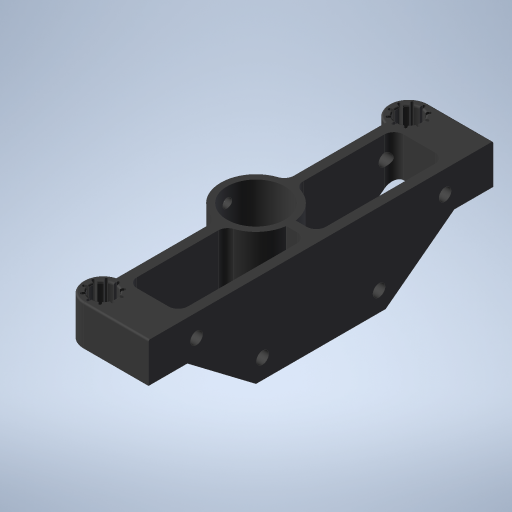
# Autodesk Inventor part: Arm Base stand
Saved by Autodesk Inventor 2024 (Build 280153000, 153)
## iProperties
Created: 2024-03-27
Part Number: Arm Base stand
Material: Generic
Document SubType Name: Modeling
Designer: drew
Density: 1 g/cm^3
Appearance: Default
Author: drew
Autodesk Inventor part; units mm, degrees
ref_plane "YZ Plane" through (0, 0, 0) normal (1, 0, 0) x (0, 1, 0)
ref_plane "XZ Plane" through (0, 0, 0) normal (0, 1, 0) x (-1, 0, 0)
ref_plane "XY Plane" through (0, 0, 0) normal (0, 0, 1) x (1, 0, 0)
sketch "Sketch1" plane through (0, 0, 0) normal (0, 1, 0) x (-1, 0, 0)
  circle A0 centre (0, 0) radius 11.43
  line L0 (-18.025, 21.2) -> (18.025, 21.2)
  line L1 (21.2, 18.025) -> (21.2, -18.025)
  line L2 (18.025, -21.2) -> (-18.025, -21.2)
  line L3 (-21.2, -18.025) -> (-21.2, 18.025)
  line L4 (-21.2, 21.2) -> (21.2, -21.2) construction
  line L5 (21.2, 21.2) -> (-21.2, -21.2) construction
  line L6 (21.2, 0) -> (-21.2, 0) construction
  line L7 (0, -21.2) -> (0, 21.2) construction
  circle A1 centre (15.5, -15.5) radius 1.6
  circle A2 centre (15.5, 15.5) radius 1.6
  circle A3 centre (-15.5, 15.5) radius 1.6
  circle A4 centre (-15.5, -15.5) radius 1.6
  arc A5 (21.2, 18.025) -> (18.025, 21.2) centre (18.025, 18.025) ccw
  arc A6 (18.025, -21.2) -> (21.2, -18.025) centre (18.025, -18.025) ccw
  arc A7 (-21.2, -18.025) -> (-18.025, -21.2) centre (-18.025, -18.025) ccw
  arc A8 (-18.025, 21.2) -> (-21.2, 18.025) centre (-18.025, 18.025) ccw
  dimension "d0" = 22.86
  dimension "d2" = 42.4
  dimension "d3" = 3.2
  dimension "d4" = 31
  dimension "d7" = 360
  dimension "d9" = 3.175
  constraints: 16 end point, 9 centre point, 9 point on line, 8 point on circle, 8 tangent, 6 midpoint, 3 equal radius, 2 parallel, 2 perpendicular, 1 coincident, 1 horizontal, 9 other
  measures "d0" diameter of A0
  measures "d2" distance of L4.end L5.end
  measures "d3" diameter of A1
  measures "d4" diameter of A1.centre L6
  measures "d9" radius of A5
extrude "Extrusion1" add sketch "Sketch1" along normal blind 2
sketch "Sketch2" plane through (0, 2, 0) normal (0, 1, 0) x (1, 0, 0)
  line L0 (18.025, 21.2) -> (-18.025, 21.2) projected
  arc A0 (-18.025, 21.2) -> (-21.2, 18.025) centre (-18.025, 18.025) ccw projected
  line L1 (-21.2, 18.025) -> (-21.2, -18.025) projected
  arc A1 (-21.2, -18.025) -> (-18.025, -21.2) centre (-18.025, -18.025) ccw projected
  line L2 (-18.025, -21.2) -> (18.025, -21.2) projected
  arc A2 (18.025, -21.2) -> (21.2, -18.025) centre (18.025, -18.025) ccw projected
  line L3 (21.2, -18.025) -> (21.2, 18.025) projected
  arc A3 (21.2, 18.025) -> (18.025, 21.2) centre (18.025, 18.025) ccw projected
  circle A4 centre (0, 0) radius 11.43 projected
  circle A5 centre (-15.5, 15.5) radius 1.6 projected
  circle A6 centre (-15.5, -15.5) radius 1.6 projected
  circle A7 centre (15.5, -15.5) radius 1.6 projected
  circle A8 centre (15.5, 15.5) radius 1.6 projected
  circle A9 centre (-15.5, -15.5) radius 4.6
  circle A10 centre (-15.5, 15.5) radius 4.6
  circle A11 centre (15.5, 15.5) radius 4.6
  circle A12 centre (15.5, -15.5) radius 4.6
  circle A13 centre (0, 0) radius 9.5
  dimension "d12" = 3
  dimension "d13" = 3
  dimension "d14" = 3
  dimension "d15" = 3
  dimension "d16" = 19
  constraints: 5 centre point, 1 coincident
  measures "d12" radial gap between concentric circles of A6 A9
  measures "d13" radial gap between concentric circles of A5 A10
  measures "d14" radial gap between concentric circles of A8 A11
  measures "d15" radial gap between concentric circles of A7 A12
  measures "d16" diameter of A13
extrude "Extrusion2" add sketch "Sketch2" along normal blind 25 contours A3 L3 A2 L2 A1 L1 A0 L0 | A4
sketch "Sketch4" plane through (0, 27, 0) normal (0, 1, 0) x (1, 0, 0)
  circle A0 centre (0, 0) radius 9.5 projected
  circle A1 centre (-15.5, 15.5) radius 4.6 projected
  circle A2 centre (-15.5, -15.5) radius 4.6 projected
  circle A3 centre (15.5, 15.5) radius 4.6 projected
  circle A4 centre (15.5, -15.5) radius 1.6 projected
  circle A5 centre (15.5, -15.5) radius 4.6 projected
  circle A6 centre (0, -50) radius 4
  line L0 (0, 0) -> (-2.5737, 0) construction
  circle A7 centre (0, 50) radius 4
  circle A8 centre (0, -50) radius 6.35
  circle A9 centre (0, 50) radius 6.35
  arc A10 (-18.025, 21.2) -> (-21.2, 18.025) centre (-18.025, 18.025) ccw projected
  line L1 (-21.2, 18.025) -> (-21.2, -18.025) projected
  arc A11 (-21.2, -18.025) -> (-18.025, -21.2) centre (-18.025, -18.025) ccw projected
  line L2 (-18.025, -21.2) -> (18.025, -21.2) projected
  arc A12 (18.025, -21.2) -> (21.2, -18.025) centre (18.025, -18.025) ccw projected
  line L3 (21.2, -18.025) -> (21.2, 18.025) projected
  arc A13 (21.2, 18.025) -> (18.025, 21.2) centre (18.025, 18.025) ccw projected
  line L4 (18.025, 21.2) -> (-18.025, 21.2) projected
  circle A14 centre (0, 0) radius 9.5 projected
  circle A15 centre (15.5, -15.5) radius 4.6 projected
  circle A16 centre (15.5, 15.5) radius 4.6 projected
  circle A17 centre (-15.5, 15.5) radius 4.6 projected
  circle A18 centre (-15.5, -15.5) radius 4.6 projected
  line L5 (-5.7806, -52.6281) -> (-20.9153, -19.3391)
  line L6 (-20.9153, 19.3391) -> (-5.7806, 52.6281)
  arc A19 (-21.2, -18.025) -> (-18.025, -21.2) centre (-18.025, -18.025) ccw projected
  line L7 (0, -56.35) -> (21.2, -56.35)
  line L8 (21.2, -56.35) -> (21.2, 56.35)
  line L9 (21.2, 56.35) -> (0, 56.35)
  line L10 (21.2, -18.025) -> (21.2, 18.025) projected
  point P0 (21.2, 18.025)
  dimension "d19" = 8
  dimension "d20" = 50
  dimension "d21" = 12.7
  dimension "d22" = 12.7
  constraints: 12 end point, 6 point on circle, 6 tangent, 4 centre point, 3 horizontal, 2 coincident, 1 collinear, 1 point on line, 1 symmetric about line, 1 vertical alignment, 1 other
  measures "d19" diameter of A6
  measures "d20" distance of point (0, 0) A6.centre
  measures "d21" diameter of A8
  measures "d22" diameter of A9
extrude "Extrusion3" add sketch "Sketch4" along normal blind 3 contours A6 | A7 | A8 | A8 L5 A11 L2 A12 L8 L7 | A11 L1 A10 L4 A13 L3 A12 L2 | A13 L4 A10 L6 A9 L9 L8 | A9
sketch "Sketch5" plane through (0, 30, 0) normal (0, 1, 0) x (1, 0, 0)
  arc A0 (-5.7806, -52.6281) -> (0, -56.35) centre (0, -50) ccw projected
  arc A1 (0, 56.35) -> (-5.7806, 52.6281) centre (0, 50) ccw projected
  circle A2 centre (0, -50) radius 4
  circle A3 centre (0, 50) radius 4
  point P0 (0, 0)
  dimension "d25" = 8
  dimension "d26" = 8
  constraints: 2 centre point, 2 coincident
  measures "d25" diameter of A2
  measures "d26" diameter of A3
extrude "Extrusion4" cut sketch "Sketch5" against normal blind 3
sketch "Sketch6" plane through (0, 27, 0) normal (0, -1, 0) x (1, 0, 0)
  circle A0 centre (0, -50) radius 4 projected
  arc A1 (-5.7806, -52.6281) -> (0, -56.35) centre (0, -50) ccw projected
  circle A2 centre (0, -50) radius 6.35
  circle A3 centre (0, 50) radius 4 projected
  circle A4 centre (0, 50) radius 6.35
  arc A5 (0, 56.35) -> (-5.7806, 52.6281) centre (0, 50) ccw projected
  point P0 (0, 0)
  point P1 (0, -56.35)
  point P2 (-5.7806, -52.6281)
  constraints: 2 centre point, 2 coincident, 2 concentric
extrude "Extrusion5" add sketch "Sketch6" along normal blind 7
sketch "Sketch7" plane through (0, 20, 50) normal (0, -1, 0) x (1, 0, 0)
  circle A0 centre (0, 0) radius 6.35 projected
  circle A1 centre (0, -100) radius 6.35 projected
  point P0 (0, -50)
extrude "Extrusion6" add sketch "Sketch7" along normal blind 3
sketch "Sketch8" plane through (0, 17, 50) normal (0, -1, 0) x (1, 0, 0)
  circle A0 centre (0, 0) radius 6.35 projected
  line L0 (0, 5) -> (0, -5) construction
  line L1 (-0.5, 5) -> (-0.5, -5)
  line L2 (0.5, -5) -> (0.5, 5)
  arc A1 (0.5, 5) -> (-0.5, 5) centre (0, 5) ccw
  arc A2 (-0.5, -5) -> (0.5, -5) centre (0, -5) ccw
  line L3 (-2.9389, 4.0451) -> (2.9389, -4.0451) construction
  line L4 (-3.3434, 3.7512) -> (2.5344, -4.339)
  line L5 (3.3434, -3.7512) -> (-2.5344, 4.339)
  arc A3 (-2.5344, 4.339) -> (-3.3434, 3.7512) centre (-2.9389, 4.0451) ccw
  arc A4 (2.5344, -4.339) -> (3.3434, -3.7512) centre (2.9389, -4.0451) ccw
  line L6 (-4.7553, 1.5451) -> (4.7553, -1.5451) construction
  line L7 (-4.9098, 1.0696) -> (4.6008, -2.0206)
  line L8 (4.9098, -1.0696) -> (-4.6008, 2.0206)
  arc A5 (-4.6008, 2.0206) -> (-4.9098, 1.0696) centre (-4.7553, 1.5451) ccw
  arc A6 (4.6008, -2.0206) -> (4.9098, -1.0696) centre (4.7553, -1.5451) ccw
  line L9 (-4.7553, -1.5451) -> (4.7553, 1.5451) construction
  line L10 (-4.6008, -2.0206) -> (4.9098, 1.0696)
  line L11 (4.6008, 2.0206) -> (-4.9098, -1.0696)
  arc A7 (-4.9098, -1.0696) -> (-4.6008, -2.0206) centre (-4.7553, -1.5451) ccw
  arc A8 (4.9098, 1.0696) -> (4.6008, 2.0206) centre (4.7553, 1.5451) ccw
  line L12 (-2.9389, -4.0451) -> (2.9389, 4.0451) construction
  line L13 (-2.5344, -4.339) -> (3.3434, 3.7512)
  line L14 (2.5344, 4.339) -> (-3.3434, -3.7512)
  arc A9 (-3.3434, -3.7512) -> (-2.5344, -4.339) centre (-2.9389, -4.0451) ccw
  arc A10 (3.3434, 3.7512) -> (2.5344, 4.339) centre (2.9389, 4.0451) ccw
  line L15 (0, -5) -> (0, 5) construction
  line L16 (0.5, -5) -> (0.5, 5)
  line L17 (-0.5, 5) -> (-0.5, -5)
  arc A11 (-0.5, -5) -> (0.5, -5) centre (0, -5) ccw
  arc A12 (0.5, 5) -> (-0.5, 5) centre (0, 5) ccw
  line L18 (0, -50) -> (2.9389, -50)
  circle A13 centre (0, -100) radius 6.35
  line L19 (0, -105) -> (0, -95) construction
  line L20 (-0.5, -105) -> (-0.5, -95)
  line L21 (0.5, -95) -> (0.5, -105)
  arc A14 (-0.5, -105) -> (0.5, -105) centre (0, -105) ccw
  arc A15 (0.5, -95) -> (-0.5, -95) centre (0, -95) ccw
  line L22 (-2.9389, -104.0451) -> (2.9389, -95.9549) construction
  line L23 (-3.3434, -103.7512) -> (2.5344, -95.661)
  line L24 (3.3434, -96.2488) -> (-2.5344, -104.339)
  arc A16 (-3.3434, -103.7512) -> (-2.5344, -104.339) centre (-2.9389, -104.0451) ccw
  arc A17 (3.3434, -96.2488) -> (2.5344, -95.661) centre (2.9389, -95.9549) ccw
  line L25 (-4.7553, -101.5451) -> (4.7553, -98.4549) construction
  line L26 (-4.9098, -101.0696) -> (4.6008, -97.9794)
  line L27 (4.9098, -98.9304) -> (-4.6008, -102.0206)
  arc A18 (-4.9098, -101.0696) -> (-4.6008, -102.0206) centre (-4.7553, -101.5451) ccw
  arc A19 (4.9098, -98.9304) -> (4.6008, -97.9794) centre (4.7553, -98.4549) ccw
  line L28 (-4.7553, -98.4549) -> (4.7553, -101.5451) construction
  line L29 (-4.6008, -97.9794) -> (4.9098, -101.0696)
  line L30 (4.6008, -102.0206) -> (-4.9098, -98.9304)
  arc A20 (-4.6008, -97.9794) -> (-4.9098, -98.9304) centre (-4.7553, -98.4549) ccw
  arc A21 (4.6008, -102.0206) -> (4.9098, -101.0696) centre (4.7553, -101.5451) ccw
  line L31 (-2.9389, -95.9549) -> (2.9389, -104.0451) construction
  line L32 (-2.5344, -95.661) -> (3.3434, -103.7512)
  line L33 (2.5344, -104.339) -> (-3.3434, -96.2488)
  arc A22 (-2.5344, -95.661) -> (-3.3434, -96.2488) centre (-2.9389, -95.9549) ccw
  arc A23 (2.5344, -104.339) -> (3.3434, -103.7512) centre (2.9389, -104.0451) ccw
  line L34 (0, -95) -> (0, -105) construction
  line L35 (0.5, -95) -> (0.5, -105)
  line L36 (-0.5, -105) -> (-0.5, -95)
  arc A24 (0.5, -95) -> (-0.5, -95) centre (0, -95) ccw
  arc A25 (-0.5, -105) -> (0.5, -105) centre (0, -105) ccw
  point P0 (-0.5, -1.5388)
  point P1 (0.5, -1.5388)
  point P2 (1.309, -0.9511)
  point P3 (1.618, 0)
  point P4 (1.309, 0.9511)
  point P5 (0.5, 1.5388)
  point P6 (-0.5, 1.5388)
  point P7 (-1.309, 0.9511)
  point P8 (-1.618, 0)
  point P9 (-1.309, -0.9511)
  point P10 (-0.5, -101.5388)
  point P11 (-0.5, -105)
  point P12 (0.5, -105)
  point P13 (0.5, -101.5388)
  point P14 (1.309, -100.9511)
  point P15 (1.618, -100)
  point P16 (1.309, -99.0489)
  point P17 (0.5, -98.4612)
  point P18 (0.5, -95)
  point P19 (-0.5, -95)
  point P20 (-0.5, -98.4612)
  point P21 (-1.309, -99.0489)
  point P22 (-1.618, -100)
  point P23 (-1.309, -100.9511)
  dimension "d33" = 10
  dimension "d34" = 0.5
  dimension "d37" = 180
  constraints: 98 end point, 48 point on circle, 37 symmetric about line, 25 centre point, 4 tangent, 1 horizontal, 1 midpoint, 1 parallel, 1 vertical, 69 other
  measures "d33" distance of L0.start L0.end
  measures "d34" radius of A2
extrude "Extrusion7" cut sketch "Sketch8" against normal through all contours A1 L2 L14 L5 L1 | L5 L14 L8 L1 | L1 L8 L4 A3 L5 | L8 L14 L11 L1 | L1 L11 L4 L8 | L14 L2 L11 L5 | L5 L11 L8 L14 | L14 A10 L13 L11 L2 | L11 L14 L1 | L1 L14 L4 L11 | L8 L11 L14 | L4 L11 L7 A5 L8 | L11 L2 L8 L5 | L5 L8 L11 | L11 L13 L8 L2 | L14 L11 L8 L5 L2 L13 L10 L7 L4 L1 | L1 L4 L14 | L4 L14 L7 L11 | L8 L2 L5 | L8 L13 L5 L2 | L11 A8 L10 L8 L13 | L4 L7 L1 | L1 L7 L14 L4 | L7 L14 L10 A7 L11 | L5 L13 L2 | L8 L10 L5 L13 | L7 L4 L10 L1 | L1 L10 L14 L7 | L7 L10 L4 | L13 L5 L10 L2 | L2 L10 L13 | L8 A6 L7 L5 L10 | L10 L4 L13 L1 | L1 L13 A9 L14 L10 | L10 L7 L13 L4 | L10 L13 L7 | L10 L5 L7 L2 | L2 L7 L13 L10 | L13 L4 L2 A2 L1 | L13 L7 L2 L4 | L7 L5 A4 L4 L2 | L20 L24 L33 L21 A14 | L24 A16 L23 L27 L20 | L20 L27 L33 L24 | L27 L23 L30 L20 | L20 L30 L33 L27 | L33 L27 L30 L24 | L24 L30 L21 L33 | L21 L30 L32 A23 L33 | L30 L23 L33 L20 | L20 L33 L30 | L33 L30 L27 | L27 A18 L26 L30 L23 | L30 L27 L24 | L24 L27 L21 L30 | L21 L27 L32 L30 | L33 L23 L20 | L20 L23 L26 L29 L32 L21 L24 L27 L30 L33 | L30 L26 L33 L23 | L24 L21 L27 | L21 L24 L32 L27 | L32 L27 L29 A21 L30 | L23 L33 L26 L20 | L20 L26 L23 | L30 A20 L29 L33 L26 | L21 L32 L24 | L32 L24 L29 L27 | L26 L33 L29 L20 | L20 L29 L23 L26 | L23 L29 L26 | L32 L29 L21 | L21 L29 L24 L32 | L29 L24 L26 A19 L27 | L29 L33 A22 L32 L20 | L20 L32 L23 L29 | L23 L32 L26 L29 | L26 L32 L29 | L29 L32 L26 L21 | L21 L26 L24 L29 | L20 A15 L21 L23 L32 | L23 L21 L26 L32 | L21 L23 A17 L24 L26
ref_plane "Work Plane2" through (0, 0, 0) normal (1, 0, 0) x (0, 1, 0)
sketch "Sketch11" plane through (0, 0, 0) normal (1, 0, 0) x (0, 1, 0)
  line L0 (17, -43.65) -> (27, -43.65) projected
  line L1 (27, -52.6281) -> (27, -19.3391) projected
  line L2 (0, -21.2) -> (27, -21.2) projected
  line L3 (0, 21.2) -> (27, 21.2) projected
  line L4 (27, 19.3391) -> (27, 52.6281) projected
  line L5 (17, 43.65) -> (27, 43.65) projected
  line L6 (17, 43.65) -> (0, 21.2)
  line L7 (0, -21.2) -> (17, -43.65)
  line L8 (17, -43.65) -> (27, -43.65)
  line L9 (27, -43.65) -> (27, -44.15)
  line L10 (27, -44.15) -> (17, -44.15)
  line L11 (17, -44.15) -> (17, -43.65)
  line L12 (17, 43.65) -> (27, 43.65)
  line L13 (27, 43.65) -> (27, 44.15)
  line L14 (27, 44.15) -> (17, 44.15)
  line L15 (17, 44.15) -> (17, 43.65)
  point P0 (0, 0)
  dimension "d46" = 0.5
  dimension "d47" = 0.5
  constraints: 20 end point, 4 parallel, 2 horizontal, 2 perpendicular, 2 point on line
  measures "d46" distance between parallel lines of L0 L10
  measures "d47" distance between parallel lines of L5 L14
extrude "Extrusion9" add sketch "Sketch11" along normal mid plane 3
sketch "Sketch12" plane through (0, 30, 0) normal (0, 1, 0) x (1, 0, 0)
  line L0 (4.6008, -52.0206) -> (3.6199, -51.7019) projected
  arc A0 (2.7372, -52.9168) -> (3.6199, -51.7019) centre (0, -50) ccw projected
  line L1 (2.7372, -52.9168) -> (3.3434, -53.7512) projected
  arc A1 (2.5344, -54.339) -> (3.3434, -53.7512) centre (2.9389, -54.0451) ccw projected
  line L2 (2.5344, -54.339) -> (1.9282, -53.5046) projected
  arc A2 (0.5, -53.9686) -> (1.9282, -53.5046) centre (0, -50) ccw projected
  line L3 (0.5, -53.9686) -> (0.5, -55) projected
  arc A3 (-0.5, -55) -> (0.5, -55) centre (0, -55) ccw projected
  line L4 (-0.5, -55) -> (-0.5, -53.9686) projected
  arc A4 (-1.9282, -53.5046) -> (-0.5, -53.9686) centre (0, -50) ccw projected
  line L5 (-1.9282, -53.5046) -> (-2.5344, -54.339) projected
  arc A5 (-3.3434, -53.7512) -> (-2.5344, -54.339) centre (-2.9389, -54.0451) ccw projected
  line L6 (-3.3434, -53.7512) -> (-2.7372, -52.9168) projected
  arc A6 (-3.6199, -51.7019) -> (-2.7372, -52.9168) centre (0, -50) ccw projected
  line L7 (-3.6199, -51.7019) -> (-4.6008, -52.0206) projected
  arc A7 (-4.9098, -51.0696) -> (-4.6008, -52.0206) centre (-4.7553, -51.5451) ccw projected
  line L8 (-4.9098, -51.0696) -> (-3.9289, -50.7508) projected
  arc A8 (-3.9289, -49.2492) -> (-3.9289, -50.7508) centre (0, -50) ccw projected
  line L9 (-3.9289, -49.2492) -> (-4.9098, -48.9304) projected
  arc A9 (-4.6008, -47.9794) -> (-4.9098, -48.9304) centre (-4.7553, -48.4549) ccw projected
  line L10 (-4.6008, -47.9794) -> (-3.6199, -48.2981) projected
  arc A10 (-2.7372, -47.0832) -> (-3.6199, -48.2981) centre (0, -50) ccw projected
  line L11 (-2.7372, -47.0832) -> (-3.3434, -46.2488) projected
  arc A11 (-2.5344, -45.661) -> (-3.3434, -46.2488) centre (-2.9389, -45.9549) ccw projected
  line L12 (-2.5344, -45.661) -> (-1.9282, -46.4954) projected
  arc A12 (-0.5, -46.0314) -> (-1.9282, -46.4954) centre (0, -50) ccw projected
  line L13 (-0.5, -46.0314) -> (-0.5, -45) projected
  arc A13 (0.5, -45) -> (-0.5, -45) centre (0, -45) ccw projected
  line L14 (0.5, -45) -> (0.5, -46.0314) projected
  arc A14 (1.9282, -46.4954) -> (0.5, -46.0314) centre (0, -50) ccw projected
  line L15 (1.9282, -46.4954) -> (2.5344, -45.661) projected
  arc A15 (3.3434, -46.2488) -> (2.5344, -45.661) centre (2.9389, -45.9549) ccw projected
  line L16 (3.3434, -46.2488) -> (2.7372, -47.0832) projected
  arc A16 (3.6199, -48.2981) -> (2.7372, -47.0832) centre (0, -50) ccw projected
  line L17 (3.6199, -48.2981) -> (4.6008, -47.9794) projected
  arc A17 (4.9098, -48.9304) -> (4.6008, -47.9794) centre (4.7553, -48.4549) ccw projected
  line L18 (4.9098, -48.9304) -> (3.9289, -49.2492) projected
  arc A18 (3.9289, -50.7508) -> (3.9289, -49.2492) centre (0, -50) ccw projected
  line L19 (3.9289, -50.7508) -> (4.9098, -51.0696) projected
  arc A19 (4.6008, -52.0206) -> (4.9098, -51.0696) centre (4.7553, -51.5451) ccw projected
  line L20 (2.5344, 45.661) -> (1.9282, 46.4954) projected
  arc A20 (0.5, 46.0314) -> (1.9282, 46.4954) centre (0, 50) ccw projected
  line L21 (0.5, 46.0314) -> (0.5, 45) projected
  arc A21 (-0.5, 45) -> (0.5, 45) centre (0, 45) ccw projected
  line L22 (-0.5, 45) -> (-0.5, 46.0314) projected
  arc A22 (-1.9282, 46.4954) -> (-0.5, 46.0314) centre (0, 50) ccw projected
  line L23 (-1.9282, 46.4954) -> (-2.5344, 45.661) projected
  arc A23 (-3.3434, 46.2488) -> (-2.5344, 45.661) centre (-2.9389, 45.9549) ccw projected
  line L24 (-3.3434, 46.2488) -> (-2.7372, 47.0832) projected
  arc A24 (-3.6199, 48.2981) -> (-2.7372, 47.0832) centre (0, 50) ccw projected
  line L25 (-3.6199, 48.2981) -> (-4.6008, 47.9794) projected
  arc A25 (-4.9098, 48.9304) -> (-4.6008, 47.9794) centre (-4.7553, 48.4549) ccw projected
  line L26 (-4.9098, 48.9304) -> (-3.9289, 49.2492) projected
  arc A26 (-3.9289, 50.7508) -> (-3.9289, 49.2492) centre (0, 50) ccw projected
  line L27 (-3.9289, 50.7508) -> (-4.9098, 51.0696) projected
  arc A27 (-4.6008, 52.0206) -> (-4.9098, 51.0696) centre (-4.7553, 51.5451) ccw projected
  line L28 (-4.6008, 52.0206) -> (-3.6199, 51.7019) projected
  arc A28 (-2.7372, 52.9168) -> (-3.6199, 51.7019) centre (0, 50) ccw projected
  line L29 (-2.7372, 52.9168) -> (-3.3434, 53.7512) projected
  arc A29 (-2.5344, 54.339) -> (-3.3434, 53.7512) centre (-2.9389, 54.0451) ccw projected
  line L30 (-2.5344, 54.339) -> (-1.9282, 53.5046) projected
  arc A30 (-0.5, 53.9686) -> (-1.9282, 53.5046) centre (0, 50) ccw projected
  line L31 (-0.5, 53.9686) -> (-0.5, 55) projected
  arc A31 (0.5, 55) -> (-0.5, 55) centre (0, 55) ccw projected
  line L32 (0.5, 55) -> (0.5, 53.9686) projected
  arc A32 (1.9282, 53.5046) -> (0.5, 53.9686) centre (0, 50) ccw projected
  line L33 (1.9282, 53.5046) -> (2.5344, 54.339) projected
  arc A33 (3.3434, 53.7512) -> (2.5344, 54.339) centre (2.9389, 54.0451) ccw projected
  line L34 (3.3434, 53.7512) -> (2.7372, 52.9168) projected
  arc A34 (3.6199, 51.7019) -> (2.7372, 52.9168) centre (0, 50) ccw projected
  line L35 (3.6199, 51.7019) -> (4.6008, 52.0206) projected
  arc A35 (4.9098, 51.0696) -> (4.6008, 52.0206) centre (4.7553, 51.5451) ccw projected
  line L36 (4.9098, 51.0696) -> (3.9289, 50.7508) projected
  arc A36 (3.9289, 49.2492) -> (3.9289, 50.7508) centre (0, 50) ccw projected
  line L37 (3.9289, 49.2492) -> (4.9098, 48.9304) projected
  arc A37 (4.6008, 47.9794) -> (4.9098, 48.9304) centre (4.7553, 48.4549) ccw projected
  line L38 (4.6008, 47.9794) -> (3.6199, 48.2981) projected
  arc A38 (2.7372, 47.0832) -> (3.6199, 48.2981) centre (0, 50) ccw projected
  line L39 (2.7372, 47.0832) -> (3.3434, 46.2488) projected
  arc A39 (2.5344, 45.661) -> (3.3434, 46.2488) centre (2.9389, 45.9549) ccw projected
  arc A40 (-5.7806, -52.6281) -> (0, -56.35) centre (0, -50) ccw projected
  line L40 (0, -56.35) -> (21.2, -56.35) projected
  line L41 (21.2, -56.35) -> (21.2, 56.35) projected
  line L42 (21.2, 56.35) -> (0, 56.35) projected
  arc A41 (0, 56.35) -> (-5.7806, 52.6281) centre (0, 50) ccw projected
  line L43 (-5.7806, 52.6281) -> (-20.9153, 19.3391) projected
  arc A42 (-20.9153, 19.3391) -> (-21.2, 18.025) centre (-18.025, 18.025) ccw projected
  line L44 (-21.2, 18.025) -> (-21.2, -18.025) projected
  arc A43 (-21.2, -18.025) -> (-20.9153, -19.3391) centre (-18.025, -18.025) ccw projected
  line L45 (-20.9153, -19.3391) -> (-5.7806, -52.6281) projected
  circle A44 centre (15.5, -15.5) radius 4.6 projected
  circle A45 centre (15.5, 15.5) radius 4.6 projected
  circle A46 centre (-15.5, -15.5) radius 4.6 projected
  circle A47 centre (-15.5, 15.5) radius 4.6 projected
  circle A48 centre (0, 0) radius 9.5 projected
  line L46 (1.5, -43.8297) -> (1.5, -21.2) projected
  line L47 (-1.5, -21.2) -> (-1.5, -43.8297) projected
  line L48 (1.5, 21.2) -> (1.5, 43.8297) projected
  line L49 (-1.5, 43.8297) -> (-1.5, 21.2) projected
  circle A49 centre (0, 0) radius 11.5
  circle A50 centre (0, -50) radius 6.35
  circle A51 centre (0, 50) radius 6.35
  arc A52 (0, 56.35) -> (-5.7806, 52.6281) centre (0, 50) ccw projected
  line L50 (-1.5, -21.2) -> (-1.5, 21.2)
  line L51 (1.5, 21.2) -> (1.5, -21.2)
  point P0 (1.5, 11.4018)
  point P1 (1.5, -11.4018)
  point P2 (0, -56.35)
  point P3 (-5.7806, -52.6281)
  point P4 (-1.5, -11.4018)
  point P5 (-1.5, 11.4018)
  point P6 (-5.7806, 52.6281)
  dimension "d48" = 2
  constraints: 4 end point, 3 centre point, 2 coincident, 2 concentric, 1 parallel, 1 vertical
  measures "d48" radial gap between concentric circles of A48 A49
extrude "Extrusion10" cut sketch "Sketch12" against normal up to surface (28 mm away) contours L45 A43 L44 A42 L43 A51 L49 L50 A49 L47 A50 | A50 L46 L51 A49 L48 A51 L42 L41 L40
sketch "Sketch13" plane through (1.5, 0, 0) normal (1, 0, 0) x (0, 0, -1)
  circle A0 centre (0, 25.2375) radius 1.5
  circle A1 centre (0, 9.3625) radius 1.5
  line L0 (11.4018, 30) -> (-11.4018, 30) projected
  point P0 (0, 0)
  point P1 (0, 30)
  dimension "d51" = 3
  dimension "d52" = 3
  dimension "d53" = 4.7625
  dimension "d54" = 15.875
  constraints: 2 centre point, 2 vertical alignment, 1 midpoint
  measures "d51" diameter of A0
  measures "d52" diameter of A1
  measures "d53" distance of point (0, 30) A0.centre
  measures "d54" distance of A1.centre A0.centre
extrude "Extrusion11" cut sketch "Sketch13" against normal through all
sketch "Sketch15" plane through (21.2, 0, 18.025) normal (1, 0, 0) x (0, 0, -1)
  line L0 (-25.625, 17) -> (-3.175, 0) projected
  line L1 (-3.175, 2) -> (-3.175, 0) projected
  line L2 (-3.175, 2) -> (6.6232, 2) projected
  line L3 (6.6232, 30) -> (6.6232, 2) projected
  line L4 (-25.8047, 30) -> (6.6232, 30) projected
  line L5 (-25.8047, 17) -> (-25.8047, 30) projected
  line L6 (-25.8047, 17) -> (-25.625, 17) projected
  line L7 (39.225, 0) -> (39.225, 2) projected
  line L8 (39.225, 0) -> (61.675, 17) projected
  line L9 (61.675, 17) -> (61.8547, 17) projected
  line L10 (61.8547, 30) -> (61.8547, 17) projected
  line L11 (29.4268, 30) -> (61.8547, 30) projected
  line L12 (29.4268, 30) -> (29.4268, 2) projected
  line L13 (29.4268, 2) -> (39.225, 2) projected
  line L14 (6.6232, 30) -> (29.4268, 30)
  line L15 (39.225, 0) -> (-3.175, 0)
  line L16 (-38.325, 17) -> (-38.325, 30) projected
  line L17 (-25.8047, 30) -> (-38.325, 30)
  line L18 (-38.325, 30) -> (-38.325, 17)
  line L19 (-38.325, 17) -> (-25.8047, 17)
  line L20 (-25.8047, 17) -> (-25.8047, 30)
  line L21 (61.8547, 17) -> (74.375, 17) projected
  line L22 (61.8547, 30) -> (74.375, 30)
  line L23 (74.375, 30) -> (74.375, 17)
  line L24 (74.375, 17) -> (61.8547, 17)
  line L25 (61.8547, 17) -> (61.8547, 30)
  point P0 (18.025, 0)
  constraints: 20 end point, 5 parallel, 2 collinear, 2 horizontal, 2 perpendicular, 1 point on line
extrude "Extrusion12" add sketch "Sketch15" against normal blind 3
sketch "Sketch16" plane through (0, 30, 0) normal (0, 1, 0) x (1, 0, 0)
  line L0 (21.2, 56.35) -> (21.2, -56.35) projected
  line L1 (21.2, 56.35) -> (18.2, 56.35) projected
  line L2 (18.2, -56.35) -> (18.2, 56.35) projected
  line L3 (21.2, -56.35) -> (18.2, -56.35) projected
  arc A0 (1.5, 43.8297) -> (-1.5, 43.8297) centre (0, 50) ccw projected
  line L4 (-1.5, 43.8297) -> (-1.5, 11.4018) projected
  arc A1 (-1.5, 11.4018) -> (-1.5, -11.4018) centre (0, 0) ccw projected
  line L5 (-1.5, -11.4018) -> (-1.5, -43.8297) projected
  arc A2 (-1.5, -43.8297) -> (1.5, -43.8297) centre (0, -50) ccw projected
  line L6 (1.5, -43.8297) -> (1.5, -11.4018) projected
  arc A3 (1.5, -11.4018) -> (1.5, 11.4018) centre (0, 0) ccw projected
  line L7 (1.5, 11.4018) -> (1.5, 43.8297) projected
  line L8 (4.6008, -52.0206) -> (3.6199, -51.7019) projected
  arc A4 (2.7372, -52.9168) -> (3.6199, -51.7019) centre (0, -50) ccw projected
  line L9 (2.7372, -52.9168) -> (3.3434, -53.7512) projected
  arc A5 (2.5344, -54.339) -> (3.3434, -53.7512) centre (2.9389, -54.0451) ccw projected
  line L10 (2.5344, -54.339) -> (1.9282, -53.5046) projected
  arc A6 (0.5, -53.9686) -> (1.9282, -53.5046) centre (0, -50) ccw projected
  line L11 (0.5, -53.9686) -> (0.5, -55) projected
  arc A7 (-0.5, -55) -> (0.5, -55) centre (0, -55) ccw projected
  line L12 (-0.5, -55) -> (-0.5, -53.9686) projected
  arc A8 (-1.9282, -53.5046) -> (-0.5, -53.9686) centre (0, -50) ccw projected
  line L13 (-1.9282, -53.5046) -> (-2.5344, -54.339) projected
  arc A9 (-3.3434, -53.7512) -> (-2.5344, -54.339) centre (-2.9389, -54.0451) ccw projected
  line L14 (-3.3434, -53.7512) -> (-2.7372, -52.9168) projected
  arc A10 (-3.6199, -51.7019) -> (-2.7372, -52.9168) centre (0, -50) ccw projected
  line L15 (-3.6199, -51.7019) -> (-4.6008, -52.0206) projected
  arc A11 (-4.9098, -51.0696) -> (-4.6008, -52.0206) centre (-4.7553, -51.5451) ccw projected
  line L16 (-4.9098, -51.0696) -> (-3.9289, -50.7508) projected
  arc A12 (-3.9289, -49.2492) -> (-3.9289, -50.7508) centre (0, -50) ccw projected
  line L17 (-3.9289, -49.2492) -> (-4.9098, -48.9304) projected
  arc A13 (-4.6008, -47.9794) -> (-4.9098, -48.9304) centre (-4.7553, -48.4549) ccw projected
  line L18 (-4.6008, -47.9794) -> (-3.6199, -48.2981) projected
  arc A14 (-2.7372, -47.0832) -> (-3.6199, -48.2981) centre (0, -50) ccw projected
  line L19 (-2.7372, -47.0832) -> (-3.3434, -46.2488) projected
  arc A15 (-2.5344, -45.661) -> (-3.3434, -46.2488) centre (-2.9389, -45.9549) ccw projected
  line L20 (-2.5344, -45.661) -> (-1.9282, -46.4954) projected
  arc A16 (-0.5, -46.0314) -> (-1.9282, -46.4954) centre (0, -50) ccw projected
  line L21 (-0.5, -46.0314) -> (-0.5, -45) projected
  arc A17 (0.5, -45) -> (-0.5, -45) centre (0, -45) ccw projected
  line L22 (0.5, -45) -> (0.5, -46.0314) projected
  arc A18 (1.9282, -46.4954) -> (0.5, -46.0314) centre (0, -50) ccw projected
  line L23 (1.9282, -46.4954) -> (2.5344, -45.661) projected
  arc A19 (3.3434, -46.2488) -> (2.5344, -45.661) centre (2.9389, -45.9549) ccw projected
  line L24 (3.3434, -46.2488) -> (2.7372, -47.0832) projected
  arc A20 (3.6199, -48.2981) -> (2.7372, -47.0832) centre (0, -50) ccw projected
  line L25 (3.6199, -48.2981) -> (4.6008, -47.9794) projected
  arc A21 (4.9098, -48.9304) -> (4.6008, -47.9794) centre (4.7553, -48.4549) ccw projected
  line L26 (4.9098, -48.9304) -> (3.9289, -49.2492) projected
  arc A22 (3.9289, -50.7508) -> (3.9289, -49.2492) centre (0, -50) ccw projected
  line L27 (3.9289, -50.7508) -> (4.9098, -51.0696) projected
  arc A23 (4.6008, -52.0206) -> (4.9098, -51.0696) centre (4.7553, -51.5451) ccw projected
  line L28 (2.5344, 45.661) -> (1.9282, 46.4954) projected
  arc A24 (0.5, 46.0314) -> (1.9282, 46.4954) centre (0, 50) ccw projected
  line L29 (0.5, 46.0314) -> (0.5, 45) projected
  arc A25 (-0.5, 45) -> (0.5, 45) centre (0, 45) ccw projected
  line L30 (-0.5, 45) -> (-0.5, 46.0314) projected
  arc A26 (-1.9282, 46.4954) -> (-0.5, 46.0314) centre (0, 50) ccw projected
  line L31 (-1.9282, 46.4954) -> (-2.5344, 45.661) projected
  arc A27 (-3.3434, 46.2488) -> (-2.5344, 45.661) centre (-2.9389, 45.9549) ccw projected
  line L32 (-3.3434, 46.2488) -> (-2.7372, 47.0832) projected
  arc A28 (-3.6199, 48.2981) -> (-2.7372, 47.0832) centre (0, 50) ccw projected
  line L33 (-3.6199, 48.2981) -> (-4.6008, 47.9794) projected
  arc A29 (-4.9098, 48.9304) -> (-4.6008, 47.9794) centre (-4.7553, 48.4549) ccw projected
  line L34 (-4.9098, 48.9304) -> (-3.9289, 49.2492) projected
  arc A30 (-3.9289, 50.7508) -> (-3.9289, 49.2492) centre (0, 50) ccw projected
  line L35 (-3.9289, 50.7508) -> (-4.9098, 51.0696) projected
  arc A31 (-4.6008, 52.0206) -> (-4.9098, 51.0696) centre (-4.7553, 51.5451) ccw projected
  line L36 (-4.6008, 52.0206) -> (-3.6199, 51.7019) projected
  arc A32 (-2.7372, 52.9168) -> (-3.6199, 51.7019) centre (0, 50) ccw projected
  line L37 (-2.7372, 52.9168) -> (-3.3434, 53.7512) projected
  arc A33 (-2.5344, 54.339) -> (-3.3434, 53.7512) centre (-2.9389, 54.0451) ccw projected
  line L38 (-2.5344, 54.339) -> (-1.9282, 53.5046) projected
  arc A34 (-0.5, 53.9686) -> (-1.9282, 53.5046) centre (0, 50) ccw projected
  line L39 (-0.5, 53.9686) -> (-0.5, 55) projected
  arc A35 (0.5, 55) -> (-0.5, 55) centre (0, 55) ccw projected
  line L40 (0.5, 55) -> (0.5, 53.9686) projected
  arc A36 (1.9282, 53.5046) -> (0.5, 53.9686) centre (0, 50) ccw projected
  line L41 (1.9282, 53.5046) -> (2.5344, 54.339) projected
  arc A37 (3.3434, 53.7512) -> (2.5344, 54.339) centre (2.9389, 54.0451) ccw projected
  line L42 (3.3434, 53.7512) -> (2.7372, 52.9168) projected
  arc A38 (3.6199, 51.7019) -> (2.7372, 52.9168) centre (0, 50) ccw projected
  line L43 (3.6199, 51.7019) -> (4.6008, 52.0206) projected
  arc A39 (4.9098, 51.0696) -> (4.6008, 52.0206) centre (4.7553, 51.5451) ccw projected
  line L44 (4.9098, 51.0696) -> (3.9289, 50.7508) projected
  arc A40 (3.9289, 49.2492) -> (3.9289, 50.7508) centre (0, 50) ccw projected
  line L45 (3.9289, 49.2492) -> (4.9098, 48.9304) projected
  arc A41 (4.6008, 47.9794) -> (4.9098, 48.9304) centre (4.7553, 48.4549) ccw projected
  line L46 (4.6008, 47.9794) -> (3.6199, 48.2981) projected
  arc A42 (2.7372, 47.0832) -> (3.6199, 48.2981) centre (0, 50) ccw projected
  line L47 (2.7372, 47.0832) -> (3.3434, 46.2488) projected
  arc A43 (2.5344, 45.661) -> (3.3434, 46.2488) centre (2.9389, 45.9549) ccw projected
  circle A44 centre (0, 0) radius 9.5 projected
  line L48 (0, 56.35) -> (18.2, 56.35)
  line L49 (-1.5, 43.65) -> (1.5, 43.65) projected
  line L50 (0, 43.65) -> (18.2, 43.65)
  line L51 (0, -56.35) -> (18.2, -56.35)
  line L52 (-1.5, -43.65) -> (1.5, -43.65) projected
  line L53 (0, -43.65) -> (18.2, -43.65)
  constraints: 8 end point, 2 midpoint, 2 perpendicular, 2 point on circle, 2 point on line, 1 collinear, 1 parallel
extrude "Extrusion13" add sketch "Sketch16" against normal up to surface (13 mm away) contours L2 L50 L7 A0 L48 | L51 A2 L6 L53 L2
sketch "Sketch17" plane through (0, 2, 0) normal (0, 1, 0) x (1, 0, 0)
  circle A0 centre (15.5, -15.5) radius 1.6 projected
  line L0 (18.2, -21.1952) -> (18.2, 21.1952) projected
  arc A1 (18.2, 21.1952) -> (18.025, 21.2) centre (18.025, 18.025) ccw projected
  line L1 (1.5, 21.2) -> (18.025, 21.2) projected
  line L2 (1.5, 11.4018) -> (1.5, 21.2) projected
  arc A2 (1.5, -11.4018) -> (1.5, 11.4018) centre (0, 0) ccw projected
  line L3 (1.5, -21.2) -> (1.5, -11.4018) projected
  line L4 (18.025, -21.2) -> (1.5, -21.2) projected
  arc A3 (18.025, -21.2) -> (18.2, -21.1952) centre (18.025, -18.025) ccw projected
  circle A4 centre (15.5, 15.5) radius 1.6 projected
  line L5 (18.2, 0) -> (11.5, 0)
  line L6 (18.2, -1.5) -> (11.4018, -1.5)
  line L7 (18.2, 1.5) -> (11.4018, 1.5)
  point P0 (14.8009, -1.5)
  dimension "d61" = 3
  constraints: 6 end point, 2 midpoint, 2 point on circle, 2 symmetric about line, 1 horizontal, 1 point on line
  measures "d61" diameter of point (14.801, -1.5) L5
extrude "Extrusion14" add sketch "Sketch17" along normal up to surface (28 mm away) contours L6 A2 L5 L0 | L5 A2 L7 L0
sketch "Sketch18" plane through (-1.5, 0, 0) normal (-1, 0, 0) x (0, 0, 1)
  circle A0 centre (-19.05, 6.35) radius 1.9844
  line L0 (0, 0) -> (0, 33.3261) construction
  line L1 (-18.025, 0) -> (18.025, 0) projected
  circle A1 centre (-40.6547, 22.7099) radius 1.9844
  line L2 (-19.05, 6.35) -> (-40.6547, 22.7099) construction
  line L3 (-43.65, 17) -> (-21.2, 0) projected
  line L4 (-43.8297, 17) -> (-43.8297, 30) projected
  circle A2 centre (19.05, 6.35) radius 1.9844
  circle A3 centre (40.6547, 22.7099) radius 1.9844
  dimension "d64" = 3.9688
  dimension "d65" = 19.05
  dimension "d66" = 6.35
  dimension "d67" = 3.9688
  dimension "d68" = 3.175
  constraints: 4 centre point, 4 end point, 2 symmetric about line, 1 parallel, 1 vertical, 2 other
  measures "d64" diameter of A0
  measures "d65" distance from line of L2.start L0
  measures "d66" distance from line of L1 L2.start
  measures "d67" diameter of A1
  measures "d68" distance from line of L4 L2.end
extrude "Extrusion15" cut sketch "Sketch18" against normal through all
fillet "Fillet1" radius 3.175 10 edges at (18.2, 16, 1.5) (18.2, 23.5, -43.65) (18.2, 16, -1.5) (18.2, 23.5, 43.65) (1.5, 16, -11.4018) (1.5, 23.5, 43.65) (1.5, 16, 11.4018) (1.5, 23.5, -43.65) (-1.5, 16, 11.4018) (-1.5, 16, -11.4018)
sketch "Sketch19" plane through (0, 2, 0) normal (0, -1, 0) x (1, 0, 0)
  circle A0 centre (0, 0) radius 9.5 projected
  circle A1 centre (0, 0) radius 11.43 projected
extrude "Extrusion16" add sketch "Sketch19" along normal blind 1
fillet "Fillet2" radius 0.5 27 edges at (3.2361, 30, 47.6489) (1.2361, 30, 46.1958) (-1.2361, 30, 46.1958) (-3.2361, 30, 47.6489) (-4, 30, 50) (-3.2361, 30, 52.3511) (-1.2361, 30, 53.8042) (1.2361, 30, 53.8042) (3.2361, 30, 52.3511) (3.9822, 30, 49.6229) (3.9822, 30, 50.3771) (10.6, 30, 56.35) (-6.3049, 30, 50.7554) (3.2361, 30, -52.3511) (1.2361, 30, -53.8042) (-1.2361, 30, -53.8042) (-3.2361, 30, -52.3511) (-4, 30, -50) (-3.2361, 30, -47.6489) (-1.2361, 30, -46.1958) (1.2361, 30, -46.1958) (3.2361, 30, -47.6489) (3.9822, 30, -50.3771) (3.9822, 30, -49.6229) (10.6, 30, -56.35) (-3.4376, 30, -55.3391) (-5.7101, 30, -47.2219)
body "Solid1"
